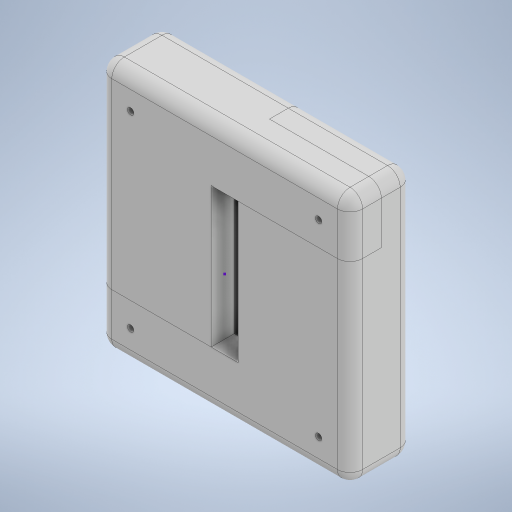
# Autodesk Inventor part: LYSO-holder
Saved by Autodesk Inventor 2023 (Build 270158000, 158)
## iProperties
Created: 2023-06-29
Part Number: LYSO-holder
Material: Generic
Document SubType Name: Modeling
Designer: AxLab
Density: 1 g/cm^3
Appearance: Default
Author: AxLab
## iProperties of the stored document LYSO-holder_3DPrint.ipt
Created: 2023-08-09
Part Number: LYSO-holder_3DPrint
Material: Generic
Document SubType Name: Modeling
Designer: AxLab
Density: 1 g/cm^3
Appearance: Default
Author: AxLab
Autodesk Inventor part; units mm, degrees
sketch "Sketch1" plane through (0, 0, 0) normal (0, 0, 1) x (1, 0, 0)
  line L0 (-20, -20) -> (20, -20)
  line L1 (20, -20) -> (20, 20)
  line L2 (20, 20) -> (-20, 20)
  line L3 (-20, 20) -> (-20, -20)
  line L4 (-20, -20) -> (20, 20) construction
  line L5 (20, -20) -> (-20, 20) construction
  point P0 (0, 0)
  dimension "d0" = 40
  dimension "d1" = 40
  constraints: 12 end point, 2 midpoint, 2 parallel, 1 horizontal, 1 perpendicular
  measures "d0" distance of L2.end L1.end
  measures "d1" distance of L1.end L0.end
extrude "Extrusion1" add sketch "Sketch1" along normal blind 10
sketch "Sketch2" plane through (0, 0, 10) normal (0, 0, 1) x (1, 0, 0)
  circle A0 centre (-15, -15) radius 0.5
  line L0 (-20, 20) -> (-20, -20) projected
  line L1 (-20, -20) -> (20, -20) projected
  point P0 (0, 0)
  dimension "d4" = 1
  dimension "d5" = 5
  dimension "d6" = 5
  constraints: 1 centre point
  measures "d4" diameter of A0
  measures "d5" distance from line of L0 A0.centre
  measures "d6" distance from line of L1 A0.centre
extrude "Extrusion2" cut sketch "Sketch2" against normal blind 10
mirror "Mirror1" about plane through (0, 0, 0) normal (1, 0, 0) of "Extrusion2"
mirror "Mirror2" about plane through (0, 0, 0) normal (0, 1, 0) of "Extrusion2", "Mirror1"
sketch "Sketch4" plane through (0, 0, 10) normal (0, 0, 1) x (1, 0, 0)
  point P0 (0, 0)
sketch "Sketch5" plane through (0, 0, 10) normal (0, 0, 1) x (1, 0, 0)
  line L0 (-2.15, -11.15) -> (2.15, -11.15)
  line L1 (2.15, -11.15) -> (2.15, 11.15)
  line L2 (2.15, 11.15) -> (-2.15, 11.15)
  line L3 (-2.15, 11.15) -> (-2.15, -11.15)
  line L4 (-2.15, -11.15) -> (2.15, 11.15) construction
  line L5 (2.15, -11.15) -> (-2.15, 11.15) construction
  point P0 (0, 0)
  dimension "d16" = 4.3
  dimension "d17" = 22.3
  constraints: 12 end point, 2 midpoint, 2 parallel, 1 horizontal, 1 perpendicular
  measures "d16" distance of L2.end L1.end
  measures "d17" distance of L1.end L0.end
extrude "Extrusion4" cut sketch "Sketch5" against normal blind 3.7
sketch "Sketch6" plane through (0, 0, 10) normal (0, 0, 1) x (1, 0, 0)
  point P0 (0, 0)
ref_plane "Work Plane1" through (0, 0, -20) normal (0, 0, -1) x (-1, 0, 0)
sketch "Sketch7" plane through (0, 0, -20) normal (0, 0, -1) x (-1, 0, 0)
  line L0 (-12.5165, 2.0003) -> (12.2108, 2.0003) construction
  line L1 (12.2108, 2.0003) -> (12.2108, -1.2478) construction
  line L2 (12.2108, -1.2478) -> (-12.5165, -1.2478) construction
  line L3 (-12.5165, -1.2478) -> (-12.5165, 2.0003) construction
  spline S0 degree 2 poles (-11.0172, -1.2379) (-11.3136, -1.2379) (-11.815, -1.0378) (-11.9978, -0.8377) knots 0 0 0 1 2 2 2
  spline S1 degree 2 poles (-11.9978, -0.8377) (-12.1806, -0.6401) (-12.3807, -0.0473) (-12.3807, 0.338) knots 0 0 0 1 2 2 2
  spline S2 degree 2 poles (-12.3807, 0.338) (-12.3807, 0.7208) (-12.1855, 1.2889) (-12.0003, 1.4989) knots 0 0 0 1 2 2 2
  spline S3 degree 2 poles (-12.0003, 1.4989) (-11.8175, 1.7039) (-11.3186, 1.9188) (-11.0098, 1.9188) knots 0 0 0 1 2 2 2
  spline S4 degree 2 poles (-11.0098, 1.9188) (-10.8567, 1.9188) (-10.5874, 1.8743) (-10.4738, 1.8398) knots 0 0 0 1 2 2 2
  spline S5 degree 2 poles (-10.4738, 1.8398) (-10.375, 1.8076) (-10.17, 1.7163) (-10.0687, 1.6619) knots 0 0 0 1 2 2 2
  line L4 (-10.0687, 1.6619) -> (-10.0687, 1.1728)
  line L5 (-10.0687, 1.1728) -> (-10.1009, 1.1728)
  spline S6 degree 2 poles (-10.1009, 1.1728) (-10.1552, 1.2222) (-10.3232, 1.3606) (-10.4442, 1.4273) knots 0 0 0 1 2 2 2
  spline S7 degree 2 poles (-10.4442, 1.4273) (-10.5603, 1.4915) (-10.8344, 1.573) (-11.0123, 1.573) knots 0 0 0 1 2 2 2
  spline S8 degree 2 poles (-11.0123, 1.573) (-11.2074, 1.573) (-11.5557, 1.4124) (-11.6866, 1.2593) knots 0 0 0 1 2 2 2
  spline S9 degree 2 poles (-11.6866, 1.2593) (-11.815, 1.1037) (-11.9583, 0.6319) (-11.9583, 0.338) knots 0 0 0 1 2 2 2
  spline S10 degree 2 poles (-11.9583, 0.338) (-11.9583, 0.0243) (-11.8076, -0.4277) (-11.6767, -0.5833) knots 0 0 0 1 2 2 2
  spline S11 degree 2 poles (-11.6767, -0.5833) (-11.5483, -0.734) (-11.2049, -0.8871) (-11.0123, -0.8871) knots 0 0 0 1 2 2 2
  spline S12 degree 2 poles (-11.0123, -0.8871) (-10.8369, -0.8871) (-10.538, -0.8007) (-10.422, -0.7365) knots 0 0 0 1 2 2 2
  spline S13 degree 2 poles (-10.422, -0.7365) (-10.3108, -0.6723) (-10.1453, -0.5389) (-10.0984, -0.4919) knots 0 0 0 1 2 2 2
  line L6 (-10.0984, -0.4919) -> (-10.0687, -0.4919)
  line L7 (-10.0687, -0.4919) -> (-10.0687, -0.9761)
  spline S14 degree 2 poles (-10.0687, -0.9761) (-10.17, -1.023) (-10.3479, -1.1094) (-10.4738, -1.149) knots 0 0 0 1 2 2 2
  spline S15 degree 2 poles (-10.4738, -1.149) (-10.6072, -1.1934) (-10.8344, -1.2379) (-11.0172, -1.2379) knots 0 0 0 1 2 2 2
  spline S16 degree 2 poles (-7.8408, -0.0399) (-7.8408, -0.6179) (-8.3965, -1.2478) (-8.8609, -1.2478) knots 0 0 0 1 2 2 2
  spline S17 degree 2 poles (-8.8609, -1.2478) (-9.3376, -1.2478) (-9.8835, -0.5982) (-9.8835, -0.0399) knots 0 0 0 1 2 2 2
  spline S18 degree 2 poles (-9.8835, -0.0399) (-9.8835, 0.5331) (-9.3203, 1.1679) (-8.8609, 1.1679) knots 0 0 0 1 2 2 2
  spline S19 degree 2 poles (-8.8609, 1.1679) (-8.3965, 1.1679) (-7.8408, 0.5356) (-7.8408, -0.0399) knots 0 0 0 1 2 2 2
  spline S20 degree 2 poles (-8.2385, -0.0399) (-8.2385, 0.4047) (-8.562, 0.8369) (-8.8609, 0.8369) knots 0 0 0 1 2 2 2
  spline S21 degree 2 poles (-8.8609, 0.8369) (-9.1598, 0.8369) (-9.4858, 0.4047) (-9.4858, -0.0399) knots 0 0 0 1 2 2 2
  spline S22 degree 2 poles (-9.4858, -0.0399) (-9.4858, -0.4722) (-9.1598, -0.9168) (-8.8609, -0.9168) knots 0 0 0 1 2 2 2
  spline S23 degree 2 poles (-8.8609, -0.9168) (-8.5645, -0.9168) (-8.2385, -0.4796) (-8.2385, -0.0399) knots 0 0 0 1 2 2 2
  spline S24 degree 2 poles (-6.8281, -1.2379) (-7.0578, -1.2379) (-7.4555, -1.1144) (-7.5864, -1.0452) knots 0 0 0 1 2 2 2
  line L8 (-7.5864, -1.0452) -> (-7.5864, -0.613)
  line L9 (-7.5864, -0.613) -> (-7.5666, -0.613)
  spline S25 degree 2 poles (-7.5666, -0.613) (-7.5172, -0.6525) (-7.3838, -0.7464) (-7.2727, -0.7982) knots 0 0 0 1 2 2 2
  spline S26 degree 2 poles (-7.2727, -0.7982) (-7.1764, -0.8452) (-6.9392, -0.9143) (-6.8133, -0.9143) knots 0 0 0 1 2 2 2
  spline S27 degree 2 poles (-6.8133, -0.9143) (-6.7219, -0.9143) (-6.5119, -0.8723) (-6.4625, -0.8377) knots 0 0 0 1 2 2 2
  spline S28 degree 2 poles (-6.4625, -0.8377) (-6.3909, -0.7908) (-6.3267, -0.6846) (-6.3267, -0.5759) knots 0 0 0 1 2 2 2
  spline S29 degree 2 poles (-6.3267, -0.5759) (-6.3267, -0.4401) (-6.4749, -0.2993) (-6.6651, -0.2524) knots 0 0 0 1 2 2 2
  spline S30 degree 2 poles (-6.6651, -0.2524) (-6.7392, -0.2351) (-6.9763, -0.1857) (-7.0776, -0.1585) knots 0 0 0 1 2 2 2
  spline S31 degree 2 poles (-7.0776, -0.1585) (-7.3394, -0.0819) (-7.5765, 0.2342) (-7.5765, 0.459) knots 0 0 0 1 2 2 2
  spline S32 degree 2 poles (-7.5765, 0.459) (-7.5765, 0.7702) (-7.1097, 1.158) (-6.7243, 1.158) knots 0 0 0 1 2 2 2
  spline S33 degree 2 poles (-6.7243, 1.158) (-6.5341, 1.158) (-6.1488, 1.0642) (-6.0179, 0.9925) knots 0 0 0 1 2 2 2
  line L10 (-6.0179, 0.9925) -> (-6.0179, 0.58)
  line L11 (-6.0179, 0.58) -> (-6.0377, 0.58)
  spline S34 degree 2 poles (-6.0377, 0.58) (-6.1859, 0.6986) (-6.5465, 0.8345) (-6.7317, 0.8345) knots 0 0 0 1 2 2 2
  spline S35 degree 2 poles (-6.7317, 0.8345) (-6.9219, 0.8345) (-7.1838, 0.6739) (-7.1838, 0.5134) knots 0 0 0 1 2 2 2
  spline S36 degree 2 poles (-7.1838, 0.5134) (-7.1838, 0.3676) (-7.0282, 0.2268) (-6.8553, 0.1824) knots 0 0 0 1 2 2 2
  spline S37 degree 2 poles (-6.8553, 0.1824) (-6.7713, 0.1601) (-6.5588, 0.1157) (-6.4428, 0.0885) knots 0 0 0 1 2 2 2
  spline S38 degree 2 poles (-6.4428, 0.0885) (-6.1908, 0.0243) (-5.9339, -0.2696) (-5.9339, -0.5241) knots 0 0 0 1 2 2 2
  spline S39 degree 2 poles (-5.9339, -0.5241) (-5.9339, -0.6723) (-6.05, -0.9341) (-6.1636, -1.0304) knots 0 0 0 1 2 2 2
  spline S40 degree 2 poles (-6.1636, -1.0304) (-6.2847, -1.1317) (-6.5934, -1.2379) (-6.8281, -1.2379) knots 0 0 0 1 2 2 2
  line L12 (-2.9823, -1.1835) -> (-2.9823, 0.1404)
  spline S41 degree 2 poles (-2.9823, 0.1404) (-2.9823, 0.2985) (-3.007, 0.5677) (-3.0465, 0.6418) knots 0 0 0 1 2 2 2
  spline S42 degree 2 poles (-3.0465, 0.6418) (-3.086, 0.7233) (-3.2367, 0.8023) (-3.3676, 0.8023) knots 0 0 0 1 2 2 2
  spline S43 degree 2 poles (-3.3676, 0.8023) (-3.4861, 0.8023) (-3.7579, 0.6566) (-3.9011, 0.5183) knots 0 0 0 1 2 2 2
  spline S44 degree 2 poles (-3.9011, 0.5183) (-3.8986, 0.4837) (-3.8937, 0.3874) (-3.8937, 0.3232) knots 0 0 0 1 2 2 2
  line L13 (-3.8937, 0.3232) -> (-3.8937, -1.1835)
  line L14 (-3.8937, -1.1835) -> (-4.279, -1.1835)
  line L15 (-4.279, -1.1835) -> (-4.279, 0.1404)
  spline S45 degree 2 poles (-4.279, 0.1404) (-4.279, 0.2985) (-4.3037, 0.5677) (-4.3432, 0.6418) knots 0 0 0 1 2 2 2
  spline S46 degree 2 poles (-4.3432, 0.6418) (-4.3828, 0.7233) (-4.5334, 0.8023) (-4.6643, 0.8023) knots 0 0 0 1 2 2 2
  spline S47 degree 2 poles (-4.6643, 0.8023) (-4.7878, 0.8023) (-5.062, 0.6467) (-5.1905, 0.5257) knots 0 0 0 1 2 2 2
  line L16 (-5.1905, 0.5257) -> (-5.1905, -1.1835)
  line L17 (-5.1905, -1.1835) -> (-5.5758, -1.1835)
  line L18 (-5.5758, -1.1835) -> (-5.5758, 1.1037)
  line L19 (-5.5758, 1.1037) -> (-5.1905, 1.1037)
  line L20 (-5.1905, 1.1037) -> (-5.1905, 0.8517)
  spline S48 degree 2 poles (-5.1905, 0.8517) (-5.0398, 1.0024) (-4.7434, 1.1679) (-4.5655, 1.1679) knots 0 0 0 1 2 2 2
  spline S49 degree 2 poles (-4.5655, 1.1679) (-4.363, 1.1679) (-4.0493, 0.9827) (-3.9678, 0.7727) knots 0 0 0 1 2 2 2
  spline S50 degree 2 poles (-3.9678, 0.7727) (-3.7924, 0.9678) (-3.4614, 1.1679) (-3.2688, 1.1679) knots 0 0 0 1 2 2 2
  spline S51 degree 2 poles (-3.2688, 1.1679) (-3.1206, 1.1679) (-2.8785, 1.0765) (-2.7896, 0.9728) knots 0 0 0 1 2 2 2
  spline S52 degree 2 poles (-2.7896, 0.9728) (-2.6982, 0.869) (-2.5969, 0.5578) (-2.5969, 0.3232) knots 0 0 0 1 2 2 2
  line L21 (-2.5969, 0.3232) -> (-2.5969, -1.1835)
  line L22 (-2.5969, -1.1835) -> (-2.9823, -1.1835)
  line L23 (-1.6633, -1.1835) -> (-2.0486, -1.1835)
  line L24 (-2.0486, -1.1835) -> (-2.0486, 1.1037)
  line L25 (-2.0486, 1.1037) -> (-1.6633, 1.1037)
  line L26 (-1.6633, 1.1037) -> (-1.6633, -1.1835)
  line L27 (-1.6361, 1.4841) -> (-2.0733, 1.4841)
  line L28 (-2.0733, 1.4841) -> (-2.0733, 1.8842)
  line L29 (-2.0733, 1.8842) -> (-1.6361, 1.8842)
  line L30 (-1.6361, 1.8842) -> (-1.6361, 1.4841)
  spline S53 degree 2 poles (-0.1887, -1.2354) (-0.4258, -1.2354) (-0.8185, -1.0897) (-0.9593, -0.9415) knots 0 0 0 1 2 2 2
  spline S54 degree 2 poles (-0.9593, -0.9415) (-1.1001, -0.7958) (-1.2557, -0.3462) (-1.2557, -0.0449) knots 0 0 0 1 2 2 2
  spline S55 degree 2 poles (-1.2557, -0.0449) (-1.2557, 0.2565) (-1.0952, 0.6961) (-0.9593, 0.8443) knots 0 0 0 1 2 2 2
  spline S56 degree 2 poles (-0.9593, 0.8443) (-0.8235, 0.995) (-0.4209, 1.1556) (-0.1887, 1.1556) knots 0 0 0 1 2 2 2
  spline S57 degree 2 poles (-0.1887, 1.1556) (-0.001, 1.1556) (0.3498, 1.0493) (0.4856, 0.9802) knots 0 0 0 1 2 2 2
  line L31 (0.4856, 0.9802) -> (0.4856, 0.5479)
  line L32 (0.4856, 0.5479) -> (0.4634, 0.5479)
  spline S58 degree 2 poles (0.4634, 0.5479) (0.4214, 0.5825) (0.293, 0.6714) (0.2016, 0.7184) knots 0 0 0 1 2 2 2
  spline S59 degree 2 poles (0.2016, 0.7184) (0.1201, 0.7579) (-0.0973, 0.8196) (-0.1961, 0.8196) knots 0 0 0 1 2 2 2
  spline S60 degree 2 poles (-0.1961, 0.8196) (-0.495, 0.8196) (-0.8581, 0.3676) (-0.8581, -0.0449) knots 0 0 0 1 2 2 2
  spline S61 degree 2 poles (-0.8581, -0.0449) (-0.8581, -0.4475) (-0.5073, -0.8995) (-0.1961, -0.8995) knots 0 0 0 1 2 2 2
  spline S62 degree 2 poles (-0.1961, -0.8995) (-0.0084, -0.8995) (0.3325, -0.7439) (0.4634, -0.6229) knots 0 0 0 1 2 2 2
  line L33 (0.4634, -0.6229) -> (0.4856, -0.6229)
  line L34 (0.4856, -0.6229) -> (0.4856, -1.0551)
  spline S63 degree 2 poles (0.4856, -1.0551) (0.4288, -1.0823) (0.2559, -1.1588) (0.1868, -1.1761) knots 0 0 0 1 2 2 2
  spline S64 degree 2 poles (0.1868, -1.1761) (0.088, -1.2058) (-0.0676, -1.2354) (-0.1887, -1.2354) knots 0 0 0 1 2 2 2
  line L35 (4.2821, 1.8645) -> (3.5163, -1.1835)
  line L36 (3.5163, -1.1835) -> (3.0619, -1.1835)
  line L37 (3.0619, -1.1835) -> (2.4419, 1.3458)
  line L38 (2.4419, 1.3458) -> (1.8392, -1.1835)
  line L39 (1.8392, -1.1835) -> (1.3897, -1.1835)
  line L40 (1.3897, -1.1835) -> (0.6116, 1.8645)
  line L41 (0.6116, 1.8645) -> (1.029, 1.8645)
  line L42 (1.029, 1.8645) -> (1.6416, -0.6624)
  line L43 (1.6416, -0.6624) -> (2.2492, 1.8645)
  line L44 (2.2492, 1.8645) -> (2.6617, 1.8645)
  line L45 (2.6617, 1.8645) -> (3.2743, -0.692)
  line L46 (3.2743, -0.692) -> (3.8844, 1.8645)
  line L47 (3.8844, 1.8645) -> (4.2821, 1.8645)
  spline S65 degree 2 poles (5.89, -0.9415) (5.8431, -0.9761) (5.685, -1.0996) (5.6109, -1.1366) knots 0 0 0 1 2 2 2
  spline S66 degree 2 poles (5.6109, -1.1366) (5.5097, -1.191) (5.3195, -1.2478) (5.1466, -1.2478) knots 0 0 0 1 2 2 2
  spline S67 degree 2 poles (5.1466, -1.2478) (5.0058, -1.2478) (4.7514, -1.1416) (4.655, -1.0452) knots 0 0 0 1 2 2 2
  spline S68 degree 2 poles (4.655, -1.0452) (4.5636, -0.9514) (4.4525, -0.6747) (4.4525, -0.5216) knots 0 0 0 1 2 2 2
  spline S69 degree 2 poles (4.4525, -0.5216) (4.4525, -0.2845) (4.6526, 0.0515) (4.8699, 0.1478) knots 0 0 0 1 2 2 2
  spline S70 degree 2 poles (4.8699, 0.1478) (5.0626, 0.2367) (5.5862, 0.3034) (5.89, 0.3207) knots 0 0 0 1 2 2 2
  line L48 (5.89, 0.3207) -> (5.89, 0.3948)
  spline S71 degree 2 poles (5.89, 0.3948) (5.89, 0.5282) (5.8085, 0.6937) (5.7344, 0.7406) knots 0 0 0 1 2 2 2
  spline S72 degree 2 poles (5.7344, 0.7406) (5.6603, 0.7875) (5.4479, 0.8172) (5.3343, 0.8172) knots 0 0 0 1 2 2 2
  spline S73 degree 2 poles (5.3343, 0.8172) (5.2009, 0.8172) (4.8403, 0.7381) (4.66, 0.6616) knots 0 0 0 1 2 2 2
  line L49 (4.66, 0.6616) -> (4.6377, 0.6616)
  line L50 (4.6377, 0.6616) -> (4.6377, 1.0543)
  spline S74 degree 2 poles (4.6377, 1.0543) (4.7439, 1.0839) (5.1416, 1.158) (5.3367, 1.158) knots 0 0 0 1 2 2 2
  spline S75 degree 2 poles (5.3367, 1.158) (5.5739, 1.158) (5.8974, 1.0839) (6.0259, 0.9876) knots 0 0 0 1 2 2 2
  spline S76 degree 2 poles (6.0259, 0.9876) (6.1519, 0.8937) (6.2754, 0.5949) (6.2754, 0.38) knots 0 0 0 1 2 2 2
  line L51 (6.2754, 0.38) -> (6.2754, -1.1835)
  line L52 (6.2754, -1.1835) -> (5.89, -1.1835)
  line L53 (5.89, -1.1835) -> (5.89, -0.9415)
  line L54 (5.89, -0.6204) -> (5.89, 0.0144)
  spline S77 degree 2 poles (5.89, 0.0144) (5.7517, 0.0021) (5.3343, -0.0399) (5.2034, -0.0794) knots 0 0 0 1 2 2 2
  spline S78 degree 2 poles (5.2034, -0.0794) (5.0502, -0.1264) (4.8502, -0.3215) (4.8502, -0.4944) knots 0 0 0 1 2 2 2
  spline S79 degree 2 poles (4.8502, -0.4944) (4.8502, -0.692) (5.0725, -0.8921) (5.2849, -0.8921) knots 0 0 0 1 2 2 2
  spline S80 degree 2 poles (5.2849, -0.8921) (5.4652, -0.8921) (5.7616, -0.7365) (5.89, -0.6204) knots 0 0 0 1 2 2 2
  spline S81 degree 2 poles (7.5079, -1.228) (7.1942, -1.228) (6.841, -0.8699) (6.841, -0.4821) knots 0 0 0 1 2 2 2
  line L55 (6.841, -0.4821) -> (6.841, 0.7851)
  line L56 (6.841, 0.7851) -> (6.5816, 0.7851)
  line L57 (6.5816, 0.7851) -> (6.5816, 1.1037)
  line L58 (6.5816, 1.1037) -> (6.841, 1.1037)
  line L59 (6.841, 1.1037) -> (6.841, 1.7607)
  line L60 (6.841, 1.7607) -> (7.2263, 1.7607)
  line L61 (7.2263, 1.7607) -> (7.2263, 1.1037)
  line L62 (7.2263, 1.1037) -> (7.9352, 1.1037)
  line L63 (7.9352, 1.1037) -> (7.9352, 0.7851)
  line L64 (7.9352, 0.7851) -> (7.2263, 0.7851)
  line L65 (7.2263, 0.7851) -> (7.2263, -0.3042)
  spline S82 degree 2 poles (7.2263, -0.3042) (7.2263, -0.4771) (7.2387, -0.6673) (7.2807, -0.7488) knots 0 0 0 1 2 2 2
  spline S83 degree 2 poles (7.2807, -0.7488) (7.3152, -0.8205) (7.4708, -0.8921) (7.6042, -0.8921) knots 0 0 0 1 2 2 2
  spline S84 degree 2 poles (7.6042, -0.8921) (7.6981, -0.8921) (7.8735, -0.8353) (7.913, -0.818) knots 0 0 0 1 2 2 2
  line L66 (7.913, -0.818) -> (7.9352, -0.818)
  line L67 (7.9352, -0.818) -> (7.9352, -1.1638)
  spline S85 degree 2 poles (7.9352, -1.1638) (7.8265, -1.1934) (7.6042, -1.228) (7.5079, -1.228) knots 0 0 0 1 2 2 2
  spline S86 degree 2 poles (9.1282, -1.2354) (8.8911, -1.2354) (8.4984, -1.0897) (8.3576, -0.9415) knots 0 0 0 1 2 2 2
  spline S87 degree 2 poles (8.3576, -0.9415) (8.2168, -0.7958) (8.0612, -0.3462) (8.0612, -0.0449) knots 0 0 0 1 2 2 2
  spline S88 degree 2 poles (8.0612, -0.0449) (8.0612, 0.2565) (8.2217, 0.6961) (8.3576, 0.8443) knots 0 0 0 1 2 2 2
  spline S89 degree 2 poles (8.3576, 0.8443) (8.4934, 0.995) (8.896, 1.1556) (9.1282, 1.1556) knots 0 0 0 1 2 2 2
  spline S90 degree 2 poles (9.1282, 1.1556) (9.3159, 1.1556) (9.6667, 1.0493) (9.8025, 0.9802) knots 0 0 0 1 2 2 2
  line L68 (9.8025, 0.9802) -> (9.8025, 0.5479)
  line L69 (9.8025, 0.5479) -> (9.7803, 0.5479)
  spline S91 degree 2 poles (9.7803, 0.5479) (9.7383, 0.5825) (9.6099, 0.6714) (9.5185, 0.7184) knots 0 0 0 1 2 2 2
  spline S92 degree 2 poles (9.5185, 0.7184) (9.437, 0.7579) (9.2196, 0.8196) (9.1208, 0.8196) knots 0 0 0 1 2 2 2
  spline S93 degree 2 poles (9.1208, 0.8196) (8.8219, 0.8196) (8.4589, 0.3676) (8.4589, -0.0449) knots 0 0 0 1 2 2 2
  spline S94 degree 2 poles (8.4589, -0.0449) (8.4589, -0.4475) (8.8096, -0.8995) (9.1208, -0.8995) knots 0 0 0 1 2 2 2
  spline S95 degree 2 poles (9.1208, -0.8995) (9.3085, -0.8995) (9.6494, -0.7439) (9.7803, -0.6229) knots 0 0 0 1 2 2 2
  line L70 (9.7803, -0.6229) -> (9.8025, -0.6229)
  line L71 (9.8025, -0.6229) -> (9.8025, -1.0551)
  spline S96 degree 2 poles (9.8025, -1.0551) (9.7457, -1.0823) (9.5728, -1.1588) (9.5037, -1.1761) knots 0 0 0 1 2 2 2
  spline S97 degree 2 poles (9.5037, -1.1761) (9.4049, -1.2058) (9.2493, -1.2354) (9.1282, -1.2354) knots 0 0 0 1 2 2 2
  line L72 (11.949, -1.1835) -> (11.5637, -1.1835)
  line L73 (11.5637, -1.1835) -> (11.5637, 0.1206)
  spline S98 degree 2 poles (11.5637, 0.1206) (11.5637, 0.2787) (11.534, 0.5504) (11.4896, 0.6319) knots 0 0 0 1 2 2 2
  spline S99 degree 2 poles (11.4896, 0.6319) (11.4426, 0.7184) (11.2747, 0.8023) (11.1314, 0.8023) knots 0 0 0 1 2 2 2
  spline S100 degree 2 poles (11.1314, 0.8023) (10.9881, 0.8023) (10.6843, 0.6492) (10.5386, 0.5257) knots 0 0 0 1 2 2 2
  line L74 (10.5386, 0.5257) -> (10.5386, -1.1835)
  line L75 (10.5386, -1.1835) -> (10.1533, -1.1835)
  line L76 (10.1533, -1.1835) -> (10.1533, 2.0003)
  line L77 (10.1533, 2.0003) -> (10.5386, 2.0003)
  line L78 (10.5386, 2.0003) -> (10.5386, 0.8493)
  spline S101 degree 2 poles (10.5386, 0.8493) (10.7115, 1.0049) (11.045, 1.1679) (11.2327, 1.1679) knots 0 0 0 1 2 2 2
  spline S102 degree 2 poles (11.2327, 1.1679) (11.5686, 1.1679) (11.949, 0.7233) (11.949, 0.3009) knots 0 0 0 1 2 2 2
  line L79 (11.949, 0.3009) -> (11.949, -1.1835)
  point P0 (0, 0)
  constraints: 2 other
emboss "Emboss1" sketch "Sketch7" operation cut depth 2 direction (0, 0, 1)
ref_plane "Work Plane2" through (-2.15, -11.15, 10) normal (1, 0, 0) x (0, 0, -1)
ref_plane "Work Plane3" through (-2.15, -11.15, 10) normal (0, 1, 0) x (1, 0, 0)
ref_plane "Work Plane4" through (2.15, -11.15, 10) normal (-1, 0, 0) x (0, 0, 1)
split body "Split14" result two bodies by plane through (2.15, -11.15, 10) normal (-1, 0, 0) first body at (-17.3163, 0.1003, 0.5)
ref_plane "Work Plane14" through (-2.15, 11.15, 6.3) normal (0, -1, 0) x (1, 0, 0)
split body "Split15" result two bodies by plane through (-2.15, 11.15, 6.3) normal (0, -1, 0) bodies 3 first body at (8.1, 3.7167, 9.5)
split body "Split16" result two bodies by plane through (-2.15, -11.15, 10) normal (0, 1, 0) bodies 2 first body at (-5.5489, 12.2483, 0.5)
ref_plane "Work Plane15" through (0, 0, 5) normal (0, 0, 1) x (1, 0, 0)
ref_plane "Work Plane16" through (0, 0, 5) normal (0, 0, 1) x (1, 0, 0)
split body "Split17" result two bodies by plane through (0, 0, 5) normal (0, 0, 1) bodies 5 first body at (6.2667, 15.3833, 5.5)
split body "Split18" result two bodies by plane through (0, 0, 5) normal (0, 0, 1) bodies 7 first body at (-3.4, -15.3833, 5.5)
combine bodies "Combine7" operation type add bodies to combine 10 4 9
combine bodies "Combine8" operation type add bodies to combine 8 6 11
fillet "Fillet20" radius 2 18 edges at (0, 20, 10) (-20, 20, 5) (-8.925, 20, 0) (-20, 0, 0) (-20, 4.425, 10) (-20, -20, 2.5) (20, 15.575, 10) (20, 20, 7.5) (-8.925, -20, 0) (-20, -15.575, 10) (0, -20, 10) (-20, -20, 7.5) (20, -20, 5) (11.075, -20, 0) (20, -4.425, 10) (20, 20, 2.5) (20, 0, 0) (11.075, 20, 0)
body "Solid34"
body "Solid36"
